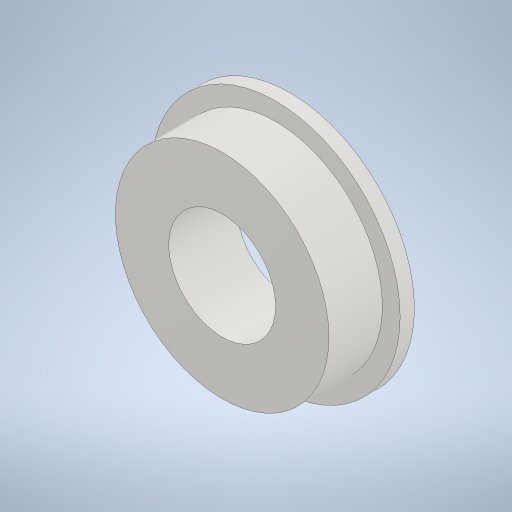
# Autodesk Inventor part: φ6φ12ベアリングa
Saved by Autodesk Inventor 2023 (Build 270158030, 158C)
## iProperties
Created: 2020-03-08
Part Number: φ6φ12ベアリングa
Material: 鋼 AISI 1006 85 HR
Document SubType Name: Modeling
Designer: happy
Density: 7.872 g/cm^3
Appearance: 鋼
Mass: 2.29995 g
Surface Area: 7.85398 cm^2
Volume: 0.292168 cm^3
Author: happy
Autodesk Inventor part; units mm, degrees
sketch "スケッチ1" plane through (0, 0, 0) normal (0, 0, 1) x (1, 0, 0)
  circle A0 centre (0, 0) radius 7
  circle A1 centre (0, 0) radius 6
  dimension "d0" = 14
  dimension "d1" = 12
  constraints: 2 centre point, 2 coincident
  measures "d0" diameter of A0
  measures "d1" diameter of A1
extrude "押し出し1" add sketch "スケッチ1" along normal blind 1
sketch "スケッチ2" plane through (0, 0, 1) normal (0, 0, 1) x (1, 0, 0)
  circle A0 centre (0, 0) radius 5.5
  circle A1 centre (0, 0) radius 3
  circle A2 centre (0, 0) radius 5
  circle A3 centre (0, 0) radius 3.5
  circle A4 centre (0, 0) radius 7 projected
  circle A5 centre (0, 0) radius 7 projected
  circle A6 centre (0, 0) radius 6 projected
  dimension "d4" = 11
  dimension "d5" = 6
  dimension "d6" = 10
  dimension "d7" = 7
  constraints: 4 centre point, 4 coincident
  measures "d4" diameter of A0
  measures "d5" diameter of A1
  measures "d6" diameter of A2
  measures "d7" diameter of A3
extrude "押し出し2" add sketch "スケッチ2" along normal blind 3 contours A3 | A6
ref_plane "作業平面1" through (0, 0, 2.5) normal (0, 0, 1) x (1, 0, 0)
sketch "スケッチ3" plane through (0, 0, 2.5) normal (0, 0, 1) x (1, 0, 0)
  circle A0 centre (0, 0) radius 6 projected
  circle A1 centre (0, 0) radius 5.5 projected
  circle A2 centre (0, 0) radius 3.5 projected
  circle A3 centre (0, 0) radius 3 projected
  circle A4 centre (4.5, 0) radius 1
  circle A5 centre (0, 0) radius 5.5 projected
  circle A6 centre (0, 0) radius 3.5 projected
  circle A7 centre (0, 0) radius 5.5 projected
  line L0 (5.5, 0) -> (3.5, 0)
  circle A8 centre (0, 0) radius 3.5 projected
  dimension "d15" = 2
  constraints: 2 end point, 2 horizontal alignment, 2 point on circle, 2 tangent, 1 centre point, 2 other
  measures "d15" diameter of A4
revolve "回転1" add sketch "スケッチ3" angle 360 about axis through (5.5, 0, 2.5) along (-1, 0, 0) picked at (4.7952, 0.1549) contours L0 A4
pattern_circular "円形状パターン1" count 6 over 360 about axis through (0, 0, -10) along (0, 0, 1) of "回転1"
ref_plane "作業平面2" through (0, 0, 3.5) normal (0, 0, 1) x (1, 0, 0)
ref_plane "作業平面3" through (0, 0, 1.5) normal (0, 0, -1) x (-1, 0, 0)
sketch "スケッチ4" plane through (0, 0, 1.5) normal (0, 0, -1) x (-1, 0, 0)
  circle A0 centre (0, 0) radius 3.5 projected
  circle A1 centre (0, 0) radius 3 projected
  circle A2 centre (0, 0) radius 6 projected
  circle A3 centre (0, 0) radius 5.5 projected
extrude "押し出し3" add sketch "スケッチ4" along normal blind 0.5 contours A3
sketch "スケッチ5" plane through (0, 0, 3.5) normal (0, 0, 1) x (1, 0, 0)
  circle A0 centre (0, 0) radius 5.5 projected
  circle A1 centre (0, 0) radius 3.5 projected
extrude "押し出し4" add sketch "スケッチ5" along normal blind 0.5
sketch "スケッチ6" plane through (0, 0, 1) normal (0, 0, -1) x (-1, 0, 0)
  circle A0 centre (0, 0) radius 6 projected
  circle A1 centre (0, 0) radius 3 projected
extrude "押し出し5" add sketch "スケッチ6" along normal blind 1
sketch "スケッチ7" plane through (0, 0, 0) normal (0, 0, -1) x (-1, 0, 0)
  circle A0 centre (0, 0) radius 3 projected
  circle A1 centre (0, 0) radius 7 projected
extrude "押し出し6" cut sketch "スケッチ7" against normal blind 0.2
